Autodesk Fusion 360 part; units mm, degrees
(part 3 of 3)
equation "d227 = rún"
equation "d228 = rún"
equation "d229 = rún"
equation "d230 = rún"
equation "d231 = biti"
equation "d232 = þykkt + biti"
equation "d233 = þykkt + lengd - biti"
equation "d234 = 4 / 3 * biti"
equation "d235 = 1 / 3 * biti"
equation "d237 = 2 / 3 * biti"
equation "d238 = 1 / 3 * biti"
equation "d239 = 10 / 3 * biti"
equation "d240 = biti"
equation "d241 = rún"
equation "d242 = 1 / 3 * biti"
equation "d243 = 1 / 3 * biti"
equation "d244 = 4 / 3 * biti"
equation "d245 = 1 / 3 * biti"
equation "d246 = rún"
equation "d247 = rún"
equation "d248 = rún"
equation "d249 = rún"
equation "d250 = rún"
equation "d251 = rún"
equation "d252 = rún"
equation "d253 = rún"
equation "d254 = rún"
equation "d255 = rún"
equation "d256 = rún"
equation "d257 = biti"
equation "d258 = þykkt + biti"
equation "d259 = þykkt + lengd - 2 * biti"
equation "d260 = biti"
equation "d261 = 1 / 3 * biti"
equation "d262 = 4 / 3 * biti"
equation "d263 = 1 / 3 * biti"
equation "d264 = 3 * biti"
equation "d265 = biti"
equation "d266 = 8 / 3 * biti"
equation "d267 = 1 / 3 * biti"
equation "d268 = 8 / 3 * biti"
equation "d269 = rún"
equation "d270 = rún"
equation "d271 = rún"
equation "d272 = rún"
equation "d273 = rún"
equation "d274 = rún"
equation "d275 = rún"
equation "d276 = rún"
equation "d277 = rún"
equation "d278 = biti"
equation "d279 = þykkt + 4 / 3 * biti"
equation "d280 = þykkt + 2 * biti"
equation "d281 = rún"
equation "d282 = 7 / 3 * biti"
equation "d283 = 1 / 3 * biti"
equation "d284 = 3 * biti"
equation "d285 = 4 / 3 * biti"
equation "d286 = 1 / 3 * biti"
equation "d287 = 1 / 3 * biti"
equation "d288 = 2 / 3 * biti"
equation "d289 = 1 / 3 * biti"
equation "d290 = 13 / 3 * biti"
equation "d291 = biti"
equation "d292 = 8 / 3 * biti"
equation "d293 = rún"
equation "d294 = rún"
equation "d295 = rún"
equation "d296 = rún"
equation "d297 = rún"
equation "d298 = rún"
equation "d299 = rún"
equation "d300 = rún"
equation "d301 = rún"
equation "d302 = rún"
equation "d303 = biti"
equation "d304 = þykkt"
equation "d305 = þykkt + 4 / 3 * biti"
equation "d306 = 13 / 3 * biti"
equation "d307 = 1 / 3 * biti"
equation "d308 = 2 / 3 * biti"
equation "d309 = 1 / 3 * biti"
equation "d310 = 1 / 3 * biti"
equation "d311 = biti"
equation "d312 = 1 / 2 * biti"
equation "d313 = 1 / 3 * biti"
equation "d314 = 1 / 3 * biti"
equation "d315 = 1 / 3 * biti"
equation "d316 = rún"
equation "d317 = rún"
equation "d318 = rún"
equation "d319 = rún"
equation "d320 = rún"
equation "d321 = rún"
equation "d322 = rún"
equation "d324 = rún"
equation "d325 = rún"
equation "d326 = rún"
equation "d327 = rún"
equation "d328 = biti"
equation "d330 = biti"
equation "d331 = þykkt"
equation "d332 = þykkt + 20 / 3 * biti"
equation "d333 = 7 / 3 * biti"
equation "d334 = 1 / 3 * biti"
equation "d335 = 2 * biti"
equation "d336 = 1 / 3 * biti"
equation "d337 = biti"
equation "d338 = biti"
equation "d339 = 3 / 2 * biti"
equation "d340 = 1 / 3 * biti"
equation "d341 = biti"
equation "d342 = 1 / 3 * biti"
equation "d343 = 17 / 6 * biti"
equation "d344 = rún"
equation "d345 = rún"
equation "d346 = rún"
equation "d347 = rún"
equation "d348 = rún"
equation "d349 = rún"
equation "d350 = rún"
equation "d351 = rún"
equation "d352 = rún"
equation "d353 = rún"
equation "d354 = rún"
equation "d355 = rún"
equation "d356 = hæð"
equation "d358 = hæð"
equation "d360 = hæð"
equation "d362 = hæð"
equation "d364 = hæð"
equation "d366 = hæð"
equation "d368 = hæð"
